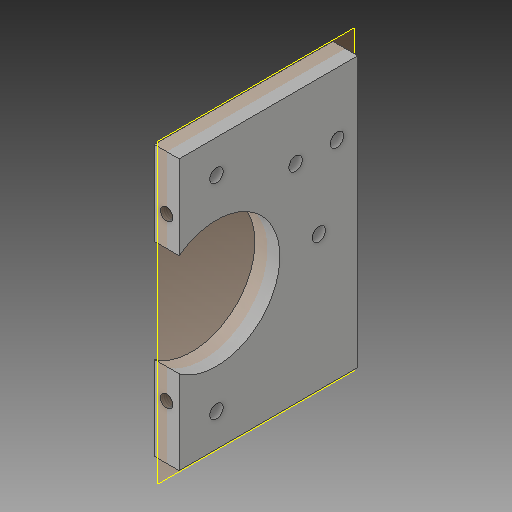
# Autodesk Inventor part: MotorHolderLongAxis
Saved by Autodesk Inventor 2018 (Build 220112000, 112)
## iProperties
Created: 2017-10-24
Part Number: MotorHolderLongAxis
Material: Generic
Document SubType Name: Modeling
Designer: m228540
Density: 1 g/cm^3
Appearance: Default
Mass: 100.573 g
Surface Area: 256.06 cm^2
Volume: 100.573 cm^3
Author: m228540
Autodesk Inventor part; units mm, degrees
ref_plane "YZ Plane" through (0, 0, 0) normal (1, 0, 0) x (0, 1, 0)
ref_plane "XZ Plane" through (0, 0, 0) normal (0, 1, 0) x (-1, 0, 0)
ref_plane "XY Plane" through (0, 0, 0) normal (0, 0, 1) x (1, 0, 0)
sketch "Sketch1" plane through (0, 0, 0) normal (1, 0, 0) x (0, 1, 0)
  line L0 (-65, 43) -> (65, 43)
  line L1 (65, 43) -> (65, -43)
  line L2 (65, -43) -> (-65, -43)
  line L3 (-65, -43) -> (-65, 43)
  line L4 (-65, 43) -> (65, -43) construction
  line L5 (65, 43) -> (-65, -43) construction
  point P0 (0, 0)
  dimension "d0" = 130
  dimension "d1" = 86
  constraints: 12 end point, 2 midpoint, 2 parallel, 1 horizontal, 1 perpendicular
  measures "d0" distance of L0.start L0.end
  measures "d1" distance of L0.end L1.end
extrude "Extrusion1" add sketch "Sketch1" along normal blind 12
sketch "Sketch2" plane through (12, 0, 0) normal (1, 0, 0) x (0, 0, -1)
  circle A0 centre (-25, 49.2145) radius 3.25
  circle A1 centre (-25, -49.2145) radius 3.25
  line L0 (-43, 65) -> (-43, -65) projected
  line L1 (-25, 49.2145) -> (-25, -49.2145) construction
  line L2 (-43, 0) -> (-25, 0) construction
  circle A2 centre (24.2145, 0) radius 3.25
  line L3 (-25, 0) -> (24.2145, 0) construction
  circle A3 centre (-25, 0) radius 30.5
  point P0 (0, 0)
  dimension "d4" = 18
  dimension "d5" = 18
  dimension "d6" = 98.429
  dimension "d7" = 6.5
  dimension "d8" = 6.5
  dimension "d9" = 6.5
  dimension "d10" = 49.2145
  dimension "d13" = 61
  constraints: 6 end point, 4 centre point, 2 horizontal, 2 midpoint, 1 coincident
  measures "d4" distance from line of L0 L1.start
  measures "d5" distance from line of L0 L1.end
  measures "d6" distance of L1.end L1.start
  measures "d7" diameter of A0
  measures "d8" diameter of A1
  measures "d9" diameter of A2
  measures "d10" distance from line of L1 L3.end
  measures "d13" diameter of A3
extrude "Extrusion2" cut sketch "Sketch2" against normal through all
ref_plane "Work Plane1" through (6, 0, 0) normal (1, 0, 0) x (0, 0, -1)
sketch "Sketch3" plane through (0, 65, 43) normal (0, 0, 1) x (1, 0, 0)
  circle A0 centre (6, -8) radius 3 construction
  circle A1 centre (6, -104) radius 3
  line L0 (0, -130) -> (12, -130) projected
  line L1 (6, -130) -> (6, 0) construction
  line L2 (0, 0) -> (12, 0) projected
  circle A2 centre (6, -26) radius 3
  point P0 (0, -65)
  dimension "d14" = 6
  dimension "d15" = 26
  dimension "d17" = 8
  dimension "d29" = 18
  constraints: 3 centre point, 3 point on line, 2 end point, 2 equal radius, 2 midpoint
  measures "d14" diameter of A0
  measures "d15" distance from line of L0 A1.centre
  measures "d17" distance from line of L2 A0.centre
  measures "d29" distance of A0.centre A2.centre
extrude "Extrusion3" cut sketch "Sketch3" against normal blind 15
sketch "Sketch4" plane through (0, -65, -43) normal (0, -1, 0) x (1, 0, 0)
  circle A0 centre (6, 15) radius 3
  circle A1 centre (6, 59) radius 3
  line L0 (0, 0) -> (12, 0) projected
  line L1 (6, 0) -> (6, 86) construction
  line L2 (0, 86) -> (12, 86) projected
  point P0 (0, 43)
  dimension "d21" = 6
  dimension "d22" = 27
  dimension "d23" = 15
  constraints: 2 centre point, 2 end point, 2 midpoint, 2 point on line, 1 equal radius
  measures "d21" diameter of A0
  measures "d22" distance from line of L2 A1.centre
  measures "d23" distance from line of L0 A0.centre
extrude "Extrusion4" cut sketch "Sketch4" against normal blind 15
sketch "Sketch6" plane through (0, 0, 0) normal (-1, 0, 0) x (0, 0, 1)
  circle A0 centre (-33, 35) radius 3 construction
  circle A1 centre (-13, 35) radius 3 construction
  circle A2 centre (-13, 35) radius 3.25
  circle A3 centre (-33, 35) radius 3.25
  point P0 (0, 0)
  dimension "d32" = 0.25
  dimension "d33" = 0.25
  constraints: 2 centre point
  measures "d32" radial gap between concentric circles of A1 A2
  measures "d33" radial gap between concentric circles of A0 A3
extrude "Extrusion6" cut sketch "Sketch6" against normal through all
thread "Thread1" size "M6x1" class "6H" standard "ANSI Metric M Profile" full length
thread "Thread2" size "M6x1" class "6H" standard "ANSI Metric M Profile" full length
thread "Thread3" size "M6x1" class "6H" standard "ANSI Metric M Profile" full length
thread "Thread4" size "M6x1" class "6H" standard "ANSI Metric M Profile" full length
equation "\"d10\" = 0.5 * d6"
body "Solid1"
